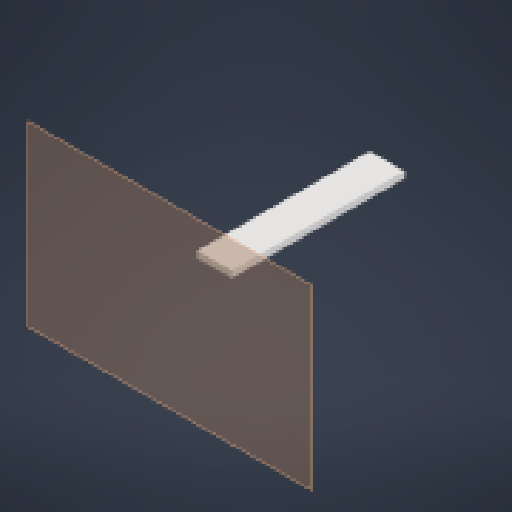
# Autodesk Inventor part: thanhdolimit
Saved by Autodesk Inventor 2023 (Build 270158000, 158)
## iProperties
Created: 2023-09-10
Part Number: thanhdolimit
Material: Generic
Document SubType Name: Modeling
Designer: philo
Density: 1 g/cm^3
Appearance: Default
Author: philo
Autodesk Inventor part; units mm, degrees
ref_plane "YZ Plane" through (0, 0, 0) normal (1, 0, 0) x (0, 1, 0)
ref_plane "XZ Plane" through (0, 0, 0) normal (0, 1, 0) x (-1, 0, 0)
ref_plane "XY Plane" through (0, 0, 0) normal (0, 0, 1) x (1, 0, 0)
ref_plane "Work Plane1" through (0, 0, 0) normal (0, 0, 1) x (1, 0, 0)
sketch "Sketch1" plane through (0, 0, 0) normal (0, 0, 1) x (1, 0, 0)
  line L0 (88.5744, 66.01) -> (72.4744, 66.01) projected
  line L1 (72.4744, 66.01) -> (88.5744, 66.01)
  line L2 (88.5744, 66.01) -> (88.5744, 63.01)
  line L3 (88.5744, 63.01) -> (72.4744, 63.01)
  line L4 (72.4744, 63.01) -> (72.4744, 66.01)
  point P0 (0, 0)
  dimension "d0" = 3
  constraints: 8 end point, 2 parallel, 1 horizontal, 1 perpendicular
  measures "d0" distance of L1.end L2.end
extrude "Extrusion1" add sketch "Sketch1" against normal blind 80
sketch "Sketch2" plane through (72.4744, 66.01, 0) normal (0, 1, 0) x (1, 0, 0)
  circle A0 centre (2.65, 28.5) radius 1.5 projected
  circle A1 centre (13.45, 28.5) radius 1.5 projected
  circle A2 centre (2.65, 43.3) radius 1.5 projected
  circle A3 centre (2.65, 62.4) radius 1.5 projected
  point P0 (-72.4744, 0)
extrude "Extrusion2" cut sketch "Sketch2" against normal blind 80
ref_plane "Work Plane2" through (0, 0, 0) normal (0, 0, 1) x (1, 0, 0)
sketch "Sketch3" plane through (0, 0, 0) normal (0, 0, 1) x (1, 0, 0)
  point P0 (0, 0)
sketch "Sketch4" plane through (72.4744, 66.01, 0) normal (0, 1, 0) x (1, 0, 0)
  line L0 (0, 0) -> (16.1, 0) projected
  line L1 (5, 0) -> (11, 0)
  line L2 (11, 0) -> (11, 7.0573)
  line L3 (11, 7.0573) -> (5, 7.0573)
  line L4 (5, 7.0573) -> (5, 0)
  line L5 (0, 0) -> (0, 80) projected
  line L6 (0, 0) -> (0, 80) projected
  line L7 (0, 0) -> (16.1, 0)
  line L8 (16.1, 0) -> (16.1, 7.0573)
  line L9 (16.1, 7.0573) -> (0, 7.0573)
  line L10 (0, 7.0573) -> (0, 0)
  point P0 (-72.4744, 0)
  point P1 (11, 7.0573)
  point P2 (11, 0)
  point P3 (5, 7.0573)
  dimension "d5" = 6
  dimension "d6" = 5
  constraints: 16 end point, 4 parallel, 2 horizontal, 2 perpendicular, 1 point on line
  measures "d5" distance of L3.end L2.end
  measures "d6" distance between parallel lines of L5 L4
extrude "Extrusion3" cut sketch "Sketch4" against normal blind 80 contours L5 L9 L4 L0 | L2 L9 L8 L0
sketch "Sketch5" plane through (72.4744, 66.01, -80) normal (0, 1, 0) x (1, 0, 0)
  circle A0 centre (8.3144, -3.4296) radius 1.5
  point P0 (-72.4744, -80)
  dimension "d9" = 3
  constraints: 1 centre point
  measures "d9" diameter of A0
extrude "Extrusion4" cut sketch "Sketch5" against normal blind 80
body "Solid1"
